Autodesk Inventor part; units mm, degrees
(part 2 of 4)
  arc A616 (35.0017, 10.0056) -> (35.1102, 10.39) centre (15.3265, 15.7621) ccw
  arc A617 (35.3927, 11.567) -> (35.4707, 11.9588) centre (15.3265, 15.7621) ccw
  arc A618 (35.66, 13.1543) -> (35.707, 13.551) centre (15.3265, 15.7621) ccw
  arc A619 (35.8019, 14.7577) -> (35.8176, 15.1569) centre (15.3265, 15.7621) ccw
  arc A620 (35.8176, 16.3673) -> (35.8019, 16.7664) centre (15.3265, 15.7621) ccw
  arc A621 (35.707, 17.9731) -> (35.66, 18.3698) centre (15.3265, 15.7621) ccw
  arc A622 (35.4707, 19.5653) -> (35.3927, 19.9571) centre (15.3265, 15.7621) ccw
  arc A623 (35.1102, 21.1341) -> (35.0017, 21.5186) centre (15.3265, 15.7621) ccw
  arc A624 (34.6277, 22.6697) -> (34.4894, 23.0445) centre (15.3265, 15.7621) ccw
  arc A625 (34.0262, 24.1628) -> (33.859, 24.5256) centre (15.3265, 15.7621) ccw
  arc A626 (33.3095, 25.6041) -> (33.1143, 25.9526) centre (15.3265, 15.7621) ccw
  arc A627 (32.4818, 26.9846) -> (32.2599, 27.3168) centre (15.3265, 15.7621) ccw
  arc A628 (31.5484, 28.296) -> (31.3011, 28.6097) centre (15.3265, 15.7621) ccw
  arc A629 (30.515, 29.5302) -> (30.2439, 29.8235) centre (15.3265, 15.7621) ccw
  arc A630 (29.388, 30.6794) -> (29.0946, 30.9505) centre (15.3265, 15.7621) ccw
  arc A631 (28.1742, 31.7366) -> (27.8605, 31.984) centre (15.3265, 15.7621) ccw
  arc A632 (26.8813, 32.6954) -> (26.5491, 32.9173) centre (15.3265, 15.7621) ccw
  arc A633 (25.5171, 33.5498) -> (25.1685, 33.745) centre (15.3265, 15.7621) ccw
  arc A634 (24.09, 34.2945) -> (23.7273, 34.4617) centre (15.3265, 15.7621) ccw
  arc A635 (22.609, 34.9249) -> (22.2342, 35.0632) centre (15.3265, 15.7621) ccw
  arc A636 (21.083, 35.4372) -> (20.6986, 35.5457) centre (15.3265, 15.7621) ccw
  arc A637 (19.5216, 35.8282) -> (19.1298, 35.9062) centre (15.3265, 15.7621) ccw
  arc A638 (17.9343, 36.0955) -> (17.5376, 36.1425) centre (15.3265, 15.7621) ccw
  arc A639 (16.3309, 36.2374) -> (15.9318, 36.2531) centre (15.3265, 15.7621) ccw
  line L0 (-7.1735, 15.7621) -> (37.8265, 15.7621)
  line L1 (15.3265, -6.7379) -> (15.3265, 38.2621)
  point P0 (0, 0)
  constraints: 960 point on circle, 480 centre point, 4 end point, 2 horizontal alignment, 2 vertical alignment, 476 other
extrude "押し出し1" add sketch "スケッチ1" along normal blind 3
sketch "スケッチ2" plane through (0, 0, 3) normal (0, 0, 1) x (1, 0, 0)
  arc A0 (15.6046, 35.4366) -> (15.5162, 35.1361) centre (20.6157, 33.7992) ccw
  arc A1 (15.5162, 35.1361) -> (15.1369, 35.1361) centre (15.3265, 15.7621) ccw
  arc A2 (15.1369, 35.1361) -> (15.0485, 35.4366) centre (10.0373, 33.7992) ccw
  arc A3 (15.0485, 35.4366) -> (14.9147, 35.8071) centre (8.9575, 33.447) ccw
  arc A4 (14.9147, 35.8071) -> (14.7213, 36.2531) centre (7.8607, 33.0129) ccw
  arc A5 (14.7213, 36.2531) -> (14.3222, 36.2374) centre (15.3265, 15.7621) ccw
  arc A6 (14.3222, 36.2374) -> (14.1644, 35.7777) centre (21.4159, 33.5455) ccw
  arc A7 (14.1644, 35.7777) -> (14.0601, 35.3977) centre (20.2884, 33.8922) ccw
  arc A8 (14.0601, 35.3977) -> (13.9955, 35.0913) centre (19.1843, 34.1586) ccw
  arc A9 (13.9955, 35.0913) -> (13.6174, 35.0615) centre (15.3265, 15.7621) ccw
  arc A10 (13.6174, 35.0615) -> (13.5057, 35.3541) centre (8.6385, 33.3286) ccw
  arc A11 (13.5057, 35.3541) -> (13.3433, 35.713) centre (7.5896, 32.8927) ccw
  arc A12 (13.3433, 35.713) -> (13.1155, 36.1425) centre (6.5302, 32.3739) ccw
  arc A13 (13.1155, 36.1425) -> (12.7188, 36.0955) centre (15.3265, 15.7621) ccw
  arc A14 (12.7188, 36.0955) -> (12.5975, 35.6248) centre (20.0019, 33.9684) ccw
  arc A15 (12.5975, 35.6248) -> (12.5234, 35.2378) centre (18.8506, 34.2256) ccw
  arc A16 (12.5234, 35.2378) -> (12.4831, 34.9273) centre (17.729, 34.4045) ccw
  arc A17 (12.4831, 34.9273) -> (12.1085, 34.8679) centre (15.3265, 15.7621) ccw
  arc A18 (12.1085, 34.8679) -> (11.9742, 35.1509) centre (7.2808, 32.7497) ccw
  arc A19 (11.9742, 35.1509) -> (11.7841, 35.4959) centre (6.2694, 32.2329) ccw
  arc A20 (11.7841, 35.4959) -> (11.5233, 35.9062) centre (5.254, 31.6326) ccw
  arc A21 (11.5233, 35.9062) -> (11.1315, 35.8282) centre (15.3265, 15.7621) ccw
  arc A22 (11.1315, 35.8282) -> (11.0475, 35.3494) centre (18.559, 34.2791) ccw
  arc A23 (11.0475, 35.3494) -> (11.0039, 34.9579) centre (17.3911, 34.4452) ccw
  arc A24 (11.0039, 34.9579) -> (10.9881, 34.6451) centre (16.2589, 34.5355) ccw
  arc A25 (10.9881, 34.6451) -> (10.6194, 34.5566) centre (15.3265, 15.7621) ccw
  arc A26 (10.6194, 34.5566) -> (10.4633, 34.8281) centre (5.9728, 32.0661) ccw
  arc A27 (10.4633, 34.8281) -> (10.2467, 35.1572) centre (5.005, 31.4715) ccw
  arc A28 (10.2467, 35.1572) -> (9.9545, 35.5457) centre (4.0399, 30.7934) ccw
  arc A29 (9.9545, 35.5457) -> (9.57, 35.4372) centre (15.3265, 15.7621) ccw
  arc A30 (9.57, 35.4372) -> (9.5239, 34.9533) centre (17.0962, 34.4756) ccw
  arc A31 (9.5239, 34.9533) -> (9.5112, 34.5595) centre (15.9189, 34.5495) ccw
  arc A32 (9.5112, 34.5595) -> (9.52, 34.2465) centre (14.7831, 34.5508) ccw
  arc A33 (9.52, 34.2465) -> (9.1593, 34.1293) centre (15.3265, 15.7621) ccw
  arc A34 (9.1593, 34.1293) -> (8.9824, 34.3877) centre (4.7224, 31.2819) ccw
  arc A35 (8.9824, 34.3877) -> (8.7406, 34.6988) centre (3.8043, 30.6133) ccw
  arc A36 (8.7406, 34.6988) -> (8.4189, 35.0632) centre (2.8953, 29.8615) ccw
  arc A37 (8.4189, 35.0632) -> (8.0441, 34.9249) centre (15.3265, 15.7621) ccw
  arc A38 (8.0441, 34.9249) -> (8.0361, 34.4389) centre (15.6225, 34.5568) ccw
  arc A39 (8.0361, 34.4389) -> (8.0543, 34.0453) centre (14.443, 34.5381) ccw
  arc A40 (8.0543, 34.0453) -> (8.0876, 33.7339) centre (13.3106, 34.4503) ccw
  arc A41 (8.0876, 33.7339) -> (7.7372, 33.5888) centre (15.3265, 15.7621) ccw
  arc A42 (7.7372, 33.5888) -> (7.5406, 33.8326) centre (3.5375, 30.4021) ccw
  arc A43 (7.5406, 33.8326) -> (7.2752, 34.1237) centre (2.6746, 29.6635) ccw
  arc A44 (7.2752, 34.1237) -> (6.9258, 34.4617) centre (1.8274, 28.8427) ccw
  arc A45 (6.9258, 34.4617) -> (6.563, 34.2945) centre (15.3265, 15.7621) ccw
  arc A46 (6.563, 34.2945) -> (6.5932, 33.8093) centre (14.147, 34.5221) ccw
  arc A47 (6.5932, 33.8093) -> (6.6422, 33.4184) centre (12.9726, 34.4109) ccw
  arc A48 (6.6422, 33.4184) -> (6.6999, 33.1106) centre (11.8506, 34.2345) ccw
  arc A49 (6.6999, 33.1106) -> (6.3619, 32.9384) centre (15.3265, 15.7621) ccw
  arc A50 (6.3619, 32.9384) -> (6.1468, 33.166) centre (2.4252, 29.432) ccw
  arc A51 (6.1468, 33.166) -> (5.8594, 33.4354) centre (1.6229, 28.628) ccw
  arc A52 (5.8594, 33.4354) -> (5.4845, 33.745) centre (0.8427, 27.7432) ccw
  arc A53 (5.4845, 33.745) -> (5.136, 33.5498) centre (15.3265, 15.7621) ccw
  arc A54 (5.136, 33.5498) -> (5.2041, 33.0685) centre (12.6787, 34.3717) ccw
  arc A55 (5.2041, 33.0685) -> (5.2837, 32.6826) centre (11.5167, 34.1687) ccw
  arc A56 (5.2837, 32.6826) -> (5.3653, 32.3803) centre (10.412, 33.9048) ccw
  arc A57 (5.3653, 32.3803) -> (5.0419, 32.1821) centre (15.3265, 15.7621) ccw
  arc A58 (5.0419, 32.1821) -> (4.8096, 32.3921) centre (1.3924, 28.3776) ccw
  arc A59 (4.8096, 32.3921) -> (4.5019, 32.6381) centre (0.6557, 27.5131) ccw
  arc A60 (4.5019, 32.6381) -> (4.104, 32.9173) centre (-0.0527, 26.5699) ccw
  arc A61 (4.104, 32.9173) -> (3.7718, 32.6954) centre (15.3265, 15.7621) ccw
  arc A62 (3.7718, 32.6954) -> (3.8775, 32.2209) centre (11.2268, 34.1066) ccw
  arc A63 (3.8775, 32.2209) -> (3.9871, 31.8425) centre (10.0843, 33.8131) ccw
  arc A64 (3.9871, 31.8425) -> (4.0922, 31.5475) centre (9.0037, 33.4633) ccw
  arc A65 (4.0922, 31.5475) -> (3.7853, 31.3246) centre (15.3265, 15.7621) ccw
  arc A66 (3.7853, 31.3246) -> (3.5372, 31.5157) centre (0.4455, 27.2455) ccw
  arc A67 (3.5372, 31.5157) -> (3.2112, 31.7368) centre (-0.221, 26.3258) ccw
  arc A68 (3.2112, 31.7368) -> (2.7926, 31.984) centre (-0.8532, 25.33) ccw
  arc A69 (2.7926, 31.984) -> (2.4789, 31.7366) centre (15.3265, 15.7621) ccw
  arc A70 (2.4789, 31.7366) -> (2.6214, 31.2719) centre (9.8001, 33.7284) ccw
  arc A71 (2.6214, 31.2719) -> (2.7604, 30.9032) centre (8.6842, 33.3461) ccw
  arc A72 (2.7604, 30.9032) -> (2.8883, 30.6174) centre (7.6343, 32.9126) ccw
  arc A73 (2.8883, 30.6174) -> (2.5999, 30.3711) centre (15.3265, 15.7621) ccw
  arc A74 (2.5999, 30.3711) -> (2.3376, 30.5421) centre (-0.4096, 26.0425) ccw
  arc A75 (2.3376, 30.5421) -> (1.9952, 30.737) centre (-1.0019, 25.0734) ccw
  arc A76 (1.9952, 30.737) -> (1.5585, 30.9505) centre (-1.554, 24.031) ccw
  arc A77 (1.5585, 30.9505) -> (1.2651, 30.6794) centre (15.3265, 15.7621) ccw
  arc A78 (1.2651, 30.6794) -> (1.4437, 30.2273) centre (8.4075, 33.2394) ccw
  arc A79 (1.4437, 30.2273) -> (1.6111, 29.8706) centre (7.325, 32.7708) ccw
  arc A80 (1.6111, 29.8706) -> (1.7611, 29.5957) centre (6.3124, 32.2563) ccw
  arc A81 (1.7611, 29.5957) -> (1.4929, 29.3275) centre (15.3265, 15.7621) ccw
  arc A82 (1.4929, 29.3275) -> (1.218, 29.4775) centre (-1.1676, 24.7762) ccw
  arc A83 (1.218, 29.4775) -> (0.8613, 29.6449) centre (-1.6821, 23.7636) ccw
  arc A84 (0.8613, 29.6449) -> (0.4092, 29.8235) centre (-2.1508, 22.6811) ccw
  arc A85 (0.4092, 29.8235) -> (0.1381, 29.5302) centre (15.3265, 15.7621) ccw
  arc A86 (0.1381, 29.5302) -> (0.3516, 29.0934) centre (7.0576, 32.6427) ccw
  arc A87 (0.3516, 29.0934) -> (0.5465, 28.751) centre (6.0152, 32.0905) ccw
  arc A88 (0.5465, 28.751) -> (0.7175, 28.4887) centre (5.0461, 31.4982) ccw
  arc A89 (0.7175, 28.4887) -> (0.4712, 28.2003) centre (15.3265, 15.7621) ccw
  arc A90 (0.4712, 28.2003) -> (0.1854, 28.3282) centre (-1.824, 23.4543) ccw
  arc A91 (0.1854, 28.3282) -> (-0.1833, 28.4672) centre (-2.2575, 22.4045) ccw
  arc A92 (-0.1833, 28.4672) -> (-0.648, 28.6097) centre (-2.6398, 21.2885) ccw
  arc A93 (-0.648, 28.6097) -> (-0.8953, 28.296) centre (15.3265, 15.7621) ccw
  arc A94 (-0.8953, 28.296) -> (-0.6482, 27.8774) centre (5.7587, 31.9418) ccw
  arc A95 (-0.6482, 27.8774) -> (-0.4271, 27.5514) centre (4.7628, 31.3096) ccw
  arc A96 (-0.4271, 27.5514) -> (-0.236, 27.3033) centre (3.8431, 30.6431) ccw
  arc A97 (-0.236, 27.3033) -> (-0.4589, 26.9964) centre (15.3265, 15.7621) ccw
  arc A98 (-0.4589, 26.9964) -> (-0.7539, 27.1015) centre (-2.3747, 22.085) ccw
  arc A99 (-0.7539, 27.1015) -> (-1.1323, 27.2111) centre (-2.7245, 21.0044) ccw
  arc A100 (-1.1323, 27.2111) -> (-1.6068, 27.3168) centre (-3.018, 19.8618) ccw
  arc A101 (-1.6068, 27.3168) -> (-1.8287, 26.9846) centre (15.3265, 15.7621) ccw
  arc A102 (-1.8287, 26.9846) -> (-1.5495, 26.5867) centre (4.5187, 31.1413) ccw
  arc A103 (-1.5495, 26.5867) -> (-1.3035, 26.279) centre (3.5755, 30.4329) ccw
  arc A104 (-1.3035, 26.279) -> (-1.0935, 26.0467) centre (2.711, 29.6962) ccw
  arc A105 (-1.0935, 26.0467) -> (-1.2916, 25.7233) centre (15.3265, 15.7621) ccw
  arc A106 (-1.2916, 25.7233) -> (-1.594, 25.8049) centre (-2.8162, 20.6766) ccw
  arc A107 (-1.594, 25.8049) -> (-1.9799, 25.8845) centre (-3.0801, 19.5719) ccw
  arc A108 (-1.9799, 25.8845) -> (-2.4612, 25.9526) centre (-3.2831, 18.4099) ccw
  arc A109 (-2.4612, 25.9526) -> (-2.6564, 25.6041) centre (15.3265, 15.7621) ccw
  arc A110 (-2.6564, 25.6041) -> (-2.3468, 25.2293) centre (3.3454, 30.2459) ccw
  arc A111 (-2.3468, 25.2293) -> (-2.0774, 24.9418) centre (2.4606, 29.4657) ccw
  arc A112 (-2.0774, 24.9418) -> (-1.8498, 24.7267) centre (1.6566, 28.6635) ccw
  arc A113 (-1.8498, 24.7267) -> (-2.022, 24.3888) centre (15.3265, 15.7621) ccw
  arc A114 (-2.022, 24.3888) -> (-2.3298, 24.4464) centre (-3.1459, 19.238) ccw
  arc A115 (-2.3298, 24.4464) -> (-2.7207, 24.4954) centre (-3.3223, 18.116) ccw
  arc A116 (-2.7207, 24.4954) -> (-3.2059, 24.5256) centre (-3.4335, 16.9417) ccw
  arc A117 (-3.2059, 24.5256) -> (-3.3731, 24.1628) centre (15.3265, 15.7621) ccw
  arc A118 (-3.3731, 24.1628) -> (-3.0351, 23.8134) centre (2.2459, 29.2612) ccw
  arc A119 (-3.0351, 23.8134) -> (-2.7439, 23.548) centre (1.4251, 28.414) ccw
  arc A120 (-2.7439, 23.548) -> (-2.5002, 23.3514) centre (0.6865, 27.5512) ccw
  arc A121 (-2.5002, 23.3514) -> (-2.6453, 23.001) centre (15.3265, 15.7621) ccw
  arc A122 (-2.6453, 23.001) -> (-2.9567, 23.0343) centre (-3.3617, 17.778) ccw
  arc A123 (-2.9567, 23.0343) -> (-3.3503, 23.0525) centre (-3.4495, 16.6456) ccw
  arc A124 (-3.3503, 23.0525) -> (-3.8363, 23.0445) centre (-3.4682, 15.4661) ccw
  arc A125 (-3.8363, 23.0445) -> (-3.9746, 22.6697) centre (15.3265, 15.7621) ccw
  arc A126 (-3.9746, 22.6697) -> (-3.6102, 22.348) centre (1.2271, 28.1933) ccw
  arc A127 (-3.6102, 22.348) -> (-3.2991, 22.1062) centre (0.4753, 27.2843) ccw
  arc A128 (-3.2991, 22.1062) -> (-3.0407, 21.9293) centre (-0.1933, 26.3662) ccw
  arc A129 (-3.0407, 21.9293) -> (-3.1579, 21.5686) centre (15.3265, 15.7621) ccw
  arc A130 (-3.1579, 21.5686) -> (-3.4709, 21.5774) centre (-3.4622, 16.3055) ccw
  arc A131 (-3.4709, 21.5774) -> (-3.8647, 21.5647) centre (-3.4609, 15.1697) ccw
  arc A132 (-3.8647, 21.5647) -> (-4.3486, 21.5186) centre (-3.387, 13.9924) ccw
  arc A133 (-4.3486, 21.5186) -> (-4.4571, 21.1341) centre (15.3265, 15.7621) ccw
  arc A134 (-4.4571, 21.1341) -> (-4.0686, 20.8419) centre (0.2952, 27.0488) ccw
  arc A135 (-4.0686, 20.8419) -> (-3.7395, 20.6253) centre (-0.3829, 26.0836) ccw
  arc A136 (-3.7395, 20.6253) -> (-3.468, 20.4692) centre (-0.9775, 25.1158) ccw
  arc A137 (-3.468, 20.4692) -> (-3.5565, 20.1005) centre (15.3265, 15.7621) ccw
  arc A138 (-3.5565, 20.1005) -> (-3.8693, 20.0847) centre (-3.4469, 14.8297) ccw
  arc A139 (-3.8693, 20.0847) -> (-4.2608, 20.0411) centre (-3.3565, 13.6975) ccw
  arc A140 (-4.2608, 20.0411) -> (-4.7396, 19.9571) centre (-3.1905, 12.5296) ccw
  arc A141 (-4.7396, 19.9571) -> (-4.8176, 19.5653) centre (15.3265, 15.7621) ccw
  arc A142 (-4.8176, 19.5653) -> (-4.4073, 19.3045) centre (-0.544, 25.8346) ccw
  arc A143 (-4.4073, 19.3045) -> (-4.0622, 19.1144) centre (-1.1443, 24.8192) ccw
  arc A144 (-4.0622, 19.1144) -> (-3.7793, 18.9801) centre (-1.6611, 23.8078) ccw
  arc A145 (-3.7793, 18.9801) -> (-3.8387, 18.6055) centre (15.3265, 15.7621) ccw
  arc A146 (-3.8387, 18.6055) -> (-4.1492, 18.5653) centre (-3.3159, 13.3596) ccw
  arc A147 (-4.1492, 18.5653) -> (-4.5362, 18.4911) centre (-3.137, 12.238) ccw
  arc A148 (-4.5362, 18.4911) -> (-5.0069, 18.3698) centre (-2.8798, 11.0868) ccw
  arc A149 (-5.0069, 18.3698) -> (-5.0539, 17.9731) centre (15.3265, 15.7621) ccw
  arc A150 (-5.0539, 17.9731) -> (-4.6244, 17.7453) centre (-1.2853, 24.5584) ccw
  arc A151 (-4.6244, 17.7453) -> (-4.2655, 17.5829) centre (-1.8041, 23.499) ccw
  arc A152 (-4.2655, 17.5829) -> (-3.9729, 17.4712) centre (-2.24, 22.4501) ccw
  arc A153 (-3.9729, 17.4712) -> (-4.0027, 17.0931) centre (15.3265, 15.7621) ccw
  arc A154 (-4.0027, 17.0931) -> (-4.3091, 17.0286) centre (-3.0699, 11.9043) ccw
  arc A155 (-4.3091, 17.0286) -> (-4.6891, 16.9243) centre (-2.8036, 10.8002) ccw
  arc A156 (-4.6891, 16.9243) -> (-5.1488, 16.7664) centre (-2.4569, 9.6727) ccw
  arc A157 (-5.1488, 16.7664) -> (-5.1645, 16.3673) centre (15.3265, 15.7621) ccw
  arc A158 (-5.1645, 16.3673) -> (-4.7185, 16.1739) centre (-1.9243, 23.2279) ccw
  arc A159 (-4.7185, 16.1739) -> (-4.348, 16.0401) centre (-2.3584, 22.1311) ccw
  arc A160 (-4.348, 16.0401) -> (-4.0475, 15.9517) centre (-2.7106, 21.0513) ccw
  arc A161 (-4.0475, 15.9517) -> (-4.0475, 15.5724) centre (15.3265, 15.7621) ccw
  arc A162 (-4.0475, 15.5724) -> (-4.348, 15.4841) centre (-2.7106, 10.4729) ccw
  arc A163 (-4.348, 15.4841) -> (-4.7185, 15.3503) centre (-2.3584, 9.3931) ccw
  arc A164 (-4.7185, 15.3503) -> (-5.1645, 15.1569) centre (-1.9243, 8.2962) ccw
  arc A165 (-5.1645, 15.1569) -> (-5.1488, 14.7577) centre (15.3265, 15.7621) ccw
  arc A166 (-5.1488, 14.7577) -> (-4.6891, 14.5999) centre (-2.4569, 21.8514) ccw
  arc A167 (-4.6891, 14.5999) -> (-4.3091, 14.4956) centre (-2.8036, 20.7239) ccw
  arc A168 (-4.3091, 14.4956) -> (-4.0027, 14.431) centre (-3.0699, 19.6198) ccw
  arc A169 (-4.0027, 14.431) -> (-3.9729, 14.053) centre (15.3265, 15.7621) ccw
  arc A170 (-3.9729, 14.053) -> (-4.2655, 13.9413) centre (-2.24, 9.074) ccw
  arc A171 (-4.2655, 13.9413) -> (-4.6244, 13.7788) centre (-1.8041, 8.0251) ccw
  arc A172 (-4.6244, 13.7788) -> (-5.0539, 13.551) centre (-1.2853, 6.9657) ccw
  arc A173 (-5.0539, 13.551) -> (-5.0069, 13.1543) centre (15.3265, 15.7621) ccw
  arc A174 (-5.0069, 13.1543) -> (-4.5362, 13.033) centre (-2.8798, 20.4374) ccw
  arc A175 (-4.5362, 13.033) -> (-4.1492, 12.9589) centre (-3.137, 19.2861) ccw
  arc A176 (-4.1492, 12.9589) -> (-3.8387, 12.9186) centre (-3.3159, 18.1645) ccw
  arc A177 (-3.8387, 12.9186) -> (-3.7793, 12.544) centre (15.3265, 15.7621) ccw
  arc A178 (-3.7793, 12.544) -> (-4.0622, 12.4097) centre (-1.6611, 7.7164) ccw
  arc A179 (-4.0622, 12.4097) -> (-4.4073, 12.2196) centre (-1.1443, 6.7049) ccw
  arc A180 (-4.4073, 12.2196) -> (-4.8176, 11.9588) centre (-0.544, 5.6895) ccw
  arc A181 (-4.8176, 11.9588) -> (-4.7396, 11.567) centre (15.3265, 15.7621) ccw
  arc A182 (-4.7396, 11.567) -> (-4.2608, 11.4831) centre (-3.1905, 18.9945) ccw
  arc A183 (-4.2608, 11.4831) -> (-3.8693, 11.4395) centre (-3.3565, 17.8266) ccw
  arc A184 (-3.8693, 11.4395) -> (-3.5565, 11.4237) centre (-3.4469, 16.6945) ccw
  arc A185 (-3.5565, 11.4237) -> (-3.468, 11.0549) centre (15.3265, 15.7621) ccw
  arc A186 (-3.468, 11.0549) -> (-3.7395, 10.8988) centre (-0.9775, 6.4083) ccw
  arc A187 (-3.7395, 10.8988) -> (-4.0686, 10.6822) centre (-0.3829, 5.4406) ccw
  arc A188 (-4.0686, 10.6822) -> (-4.4571, 10.39) centre (0.2952, 4.4754) ccw
  arc A189 (-4.4571, 10.39) -> (-4.3486, 10.0056) centre (15.3265, 15.7621) ccw
  arc A190 (-4.3486, 10.0056) -> (-3.8647, 9.9594) centre (-3.387, 17.5317) ccw
  arc A191 (-3.8647, 9.9594) -> (-3.4709, 9.9467) centre (-3.4609, 16.3544) ccw
  arc A192 (-3.4709, 9.9467) -> (-3.1579, 9.9555) centre (-3.4622, 15.2186) ccw
  arc A193 (-3.1579, 9.9555) -> (-3.0407, 9.5948) centre (15.3265, 15.7621) ccw
  arc A194 (-3.0407, 9.5948) -> (-3.2991, 9.4179) centre (-0.1933, 5.158) ccw
  arc A195 (-3.2991, 9.4179) -> (-3.6102, 9.1762) centre (0.4753, 4.2398) ccw
  arc A196 (-3.6102, 9.1762) -> (-3.9746, 8.8544) centre (1.2271, 3.3308) ccw
  arc A197 (-3.9746, 8.8544) -> (-3.8363, 8.4796) centre (15.3265, 15.7621) ccw
  arc A198 (-3.8363, 8.4796) -> (-3.3503, 8.4716) centre (-3.4682, 16.058) ccw
  arc A199 (-3.3503, 8.4716) -> (-2.9567, 8.4898) centre (-3.4495, 14.8785) ccw
  arc A200 (-2.9567, 8.4898) -> (-2.6453, 8.5231) centre (-3.3617, 13.7462) ccw
  arc A201 (-2.6453, 8.5231) -> (-2.5002, 8.1727) centre (15.3265, 15.7621) ccw
  arc A202 (-2.5002, 8.1727) -> (-2.7439, 7.9761) centre (0.6865, 3.973) ccw
  arc A203 (-2.7439, 7.9761) -> (-3.0351, 7.7107) centre (1.4251, 3.1101) ccw
  arc A204 (-3.0351, 7.7107) -> (-3.3731, 7.3613) centre (2.2459, 2.2629) ccw
  arc A205 (-3.3731, 7.3613) -> (-3.2059, 6.9986) centre (15.3265, 15.7621) ccw
  arc A206 (-3.2059, 6.9986) -> (-2.7207, 7.0287) centre (-3.4335, 14.5825) ccw
  arc A207 (-2.7207, 7.0287) -> (-2.3298, 7.0777) centre (-3.3223, 13.4081) ccw
  arc A208 (-2.3298, 7.0777) -> (-2.022, 7.1354) centre (-3.1459, 12.2861) ccw
  arc A209 (-2.022, 7.1354) -> (-1.8498, 6.7975) centre (15.3265, 15.7621) ccw
  arc A210 (-1.8498, 6.7975) -> (-2.0774, 6.5823) centre (1.6566, 2.8607) ccw
  arc A211 (-2.0774, 6.5823) -> (-2.3468, 6.2949) centre (2.4606, 2.0585) ccw
  arc A212 (-2.3468, 6.2949) -> (-2.6564, 5.9201) centre (3.3454, 1.2782) ccw
  arc A213 (-2.6564, 5.9201) -> (-2.4612, 5.5715) centre (15.3265, 15.7621) ccw
  arc A214 (-2.4612, 5.5715) -> (-1.9799, 5.6397) centre (-3.2831, 13.1142) ccw
  arc A215 (-1.9799, 5.6397) -> (-1.594, 5.7192) centre (-3.0801, 11.9522) ccw
  arc A216 (-1.594, 5.7192) -> (-1.2916, 5.8008) centre (-2.8162, 10.8475) ccw
  arc A217 (-1.2916, 5.8008) -> (-1.0935, 5.4775) centre (15.3265, 15.7621) ccw
  arc A218 (-1.0935, 5.4775) -> (-1.3035, 5.2451) centre (2.711, 1.8279) ccw
  arc A219 (-1.3035, 5.2451) -> (-1.5495, 4.9374) centre (3.5755, 1.0913) ccw
  arc A220 (-1.5495, 4.9374) -> (-1.8287, 4.5395) centre (4.5187, 0.3829) ccw
  arc A221 (-1.8287, 4.5395) -> (-1.6068, 4.2073) centre (15.3265, 15.7621) ccw
  arc A222 (-1.6068, 4.2073) -> (-1.1323, 4.313) centre (-3.018, 11.6623) ccw
  arc A223 (-1.1323, 4.313) -> (-0.7539, 4.4226) centre (-2.7245, 10.5198) ccw
  arc A224 (-0.7539, 4.4226) -> (-0.4589, 4.5277) centre (-2.3747, 9.4392) ccw
  arc A225 (-0.4589, 4.5277) -> (-0.236, 4.2209) centre (15.3265, 15.7621) ccw
  arc A226 (-0.236, 4.2209) -> (-0.4271, 3.9728) centre (3.8431, 0.8811) ccw
  arc A227 (-0.4271, 3.9728) -> (-0.6482, 3.6467) centre (4.7628, 0.2145) ccw
  arc A228 (-0.6482, 3.6467) -> (-0.8953, 3.2281) centre (5.7587, -0.4177) ccw
  arc A229 (-0.8953, 3.2281) -> (-0.648, 2.9144) centre (15.3265, 15.7621) ccw
  arc A230 (-0.648, 2.9144) -> (-0.1833, 3.057) centre (-2.6398, 10.2356) ccw
  arc A231 (-0.1833, 3.057) -> (0.1854, 3.1959) centre (-2.2575, 9.1197) ccw
  arc A232 (0.1854, 3.1959) -> (0.4712, 3.3238) centre (-1.824, 8.0698) ccw
  arc A233 (0.4712, 3.3238) -> (0.7175, 3.0354) centre (15.3265, 15.7621) ccw
  arc A234 (0.7175, 3.0354) -> (0.5465, 2.7731) centre (5.0461, 0.026) ccw
  arc A235 (0.5465, 2.7731) -> (0.3516, 2.4307) centre (6.0152, -0.5664) ccw
  arc A236 (0.3516, 2.4307) -> (0.1381, 1.994) centre (7.0576, -1.1185) ccw
  arc A237 (0.1381, 1.994) -> (0.4092, 1.7006) centre (15.3265, 15.7621) ccw
  arc A238 (0.4092, 1.7006) -> (0.8613, 1.8792) centre (-2.1508, 8.843) ccw
  arc A239 (0.8613, 1.8792) -> (1.218, 2.0467) centre (-1.6821, 7.7605) ccw
  arc A240 (1.218, 2.0467) -> (1.4929, 2.1966) centre (-1.1676, 6.7479) ccw
  arc A241 (1.4929, 2.1966) -> (1.7611, 1.9284) centre (15.3265, 15.7621) ccw
  arc A242 (1.7611, 1.9284) -> (1.6111, 1.6535) centre (6.3124, -0.7321) ccw
  arc A243 (1.6111, 1.6535) -> (1.4437, 1.2969) centre (7.325, -1.2466) ccw
  arc A244 (1.4437, 1.2969) -> (1.2651, 0.8447) centre (8.4075, -1.7153) ccw
  arc A245 (1.2651, 0.8447) -> (1.5585, 0.5736) centre (15.3265, 15.7621) ccw
  arc A246 (1.5585, 0.5736) -> (1.9952, 0.7871) centre (-1.554, 7.4931) ccw
  arc A247 (1.9952, 0.7871) -> (2.3376, 0.982) centre (-1.0019, 6.4507) ccw
  arc A248 (2.3376, 0.982) -> (2.5999, 1.1531) centre (-0.4096, 5.4816) ccw
  arc A249 (2.5999, 1.1531) -> (2.8883, 0.9068) centre (15.3265, 15.7621) ccw
  arc A250 (2.8883, 0.9068) -> (2.7604, 0.6209) centre (7.6343, -1.3885) ccw
  arc A251 (2.7604, 0.6209) -> (2.6214, 0.2522) centre (8.6842, -1.822) ccw
  arc A252 (2.6214, 0.2522) -> (2.4789, -0.2125) centre (9.8001, -2.2042) ccw
  arc A253 (2.4789, -0.2125) -> (2.7926, -0.4598) centre (15.3265, 15.7621) ccw
  arc A254 (2.7926, -0.4598) -> (3.2112, -0.2127) centre (-0.8532, 6.1942) ccw
  arc A255 (3.2112, -0.2127) -> (3.5372, 0.0085) centre (-0.221, 5.1983) ccw
  arc A256 (3.5372, 0.0085) -> (3.7853, 0.1996) centre (0.4455, 4.2787) ccw
  arc A257 (3.7853, 0.1996) -> (4.0922, -0.0233) centre (15.3265, 15.7621) ccw
  arc A258 (4.0922, -0.0233) -> (3.9871, -0.3184) centre (9.0037, -1.9392) ccw
  arc A259 (3.9871, -0.3184) -> (3.8775, -0.6968) centre (10.0843, -2.2889) ccw
  arc A260 (3.8775, -0.6968) -> (3.7718, -1.1713) centre (11.2268, -2.5825) ccw
  arc A261 (3.7718, -1.1713) -> (4.104, -1.3932) centre (15.3265, 15.7621) ccw
  arc A262 (4.104, -1.3932) -> (4.5019, -1.114) centre (-0.0527, 4.9542) ccw
  arc A263 (4.5019, -1.114) -> (4.8096, -0.868) centre (0.6557, 4.011) ccw
  arc A264 (4.8096, -0.868) -> (5.0419, -0.658) centre (1.3924, 3.1465) ccw
  arc A265 (5.0419, -0.658) -> (5.3653, -0.8561) centre (15.3265, 15.7621) ccw
  arc A266 (5.3653, -0.8561) -> (5.2837, -1.1585) centre (10.412, -2.3807) ccw
  arc A267 (5.2837, -1.1585) -> (5.2041, -1.5443) centre (11.5167, -2.6446) ccw
  arc A268 (5.2041, -1.5443) -> (5.136, -2.0257) centre (12.6787, -2.8476) ccw
  arc A269 (5.136, -2.0257) -> (5.4845, -2.2208) centre (15.3265, 15.7621) ccw
  arc A270 (5.4845, -2.2208) -> (5.8594, -1.9113) centre (0.8427, 3.7809) ccw
  arc A271 (5.8594, -1.9113) -> (6.1468, -1.6418) centre (1.6229, 2.8962) ccw
  arc A272 (6.1468, -1.6418) -> (6.3619, -1.4143) centre (2.4252, 2.0921) ccw
  arc A273 (6.3619, -1.4143) -> (6.6999, -1.5864) centre (15.3265, 15.7621) ccw
  arc A274 (6.6999, -1.5864) -> (6.6422, -1.8943) centre (11.8506, -2.7104) ccw
  arc A275 (6.6422, -1.8943) -> (6.5932, -2.2852) centre (12.9726, -2.8868) ccw
  arc A276 (6.5932, -2.2852) -> (6.563, -2.7704) centre (14.147, -2.998) ccw
  arc A277 (6.563, -2.7704) -> (6.9258, -2.9376) centre (15.3265, 15.7621) ccw
  arc A278 (6.9258, -2.9376) -> (7.2752, -2.5996) centre (1.8274, 2.6814) ccw
  arc A279 (7.2752, -2.5996) -> (7.5406, -2.3084) centre (2.6746, 1.8607) ccw
  arc A280 (7.5406, -2.3084) -> (7.7372, -2.0647) centre (3.5375, 1.122) ccw
  arc A281 (7.7372, -2.0647) -> (8.0876, -2.2098) centre (15.3265, 15.7621) ccw
  arc A282 (8.0876, -2.2098) -> (8.0543, -2.5212) centre (13.3106, -2.9261) ccw
  arc A283 (8.0543, -2.5212) -> (8.0361, -2.9148) centre (14.443, -3.014) ccw
  arc A284 (8.0361, -2.9148) -> (8.0441, -3.4008) centre (15.6225, -3.0327) ccw
  arc A285 (8.0441, -3.4008) -> (8.4189, -3.5391) centre (15.3265, 15.7621) ccw
  arc A286 (8.4189, -3.5391) -> (8.7406, -3.1747) centre (2.8953, 1.6626) ccw
  arc A287 (8.7406, -3.1747) -> (8.9824, -2.8636) centre (3.8043, 0.9109) ccw
  arc A288 (8.9824, -2.8636) -> (9.1593, -2.6052) centre (4.7224, 0.2422) ccw
  arc A289 (9.1593, -2.6052) -> (9.52, -2.7224) centre (15.3265, 15.7621) ccw
  arc A290 (9.52, -2.7224) -> (9.5112, -3.0354) centre (14.7831, -3.0267) ccw
  arc A291 (9.5112, -3.0354) -> (9.5239, -3.4292) centre (15.9189, -3.0254) ccw
  arc A292 (9.5239, -3.4292) -> (9.57, -3.9131) centre (17.0962, -2.9515) ccw
  arc A293 (9.57, -3.9131) -> (9.9545, -4.0215) centre (15.3265, 15.7621) ccw
  arc A294 (9.9545, -4.0215) -> (10.2467, -3.633) centre (4.0399, 0.7308) ccw
  arc A295 (10.2467, -3.633) -> (10.4633, -3.3039) centre (5.005, 0.0526) ccw
  arc A296 (10.4633, -3.3039) -> (10.6194, -3.0324) centre (5.9728, -0.5419) ccw
  arc A297 (10.6194, -3.0324) -> (10.9881, -3.121) centre (15.3265, 15.7621) ccw
  arc A298 (10.9881, -3.121) -> (11.0039, -3.4337) centre (16.2589, -3.0114) ccw
  arc A299 (11.0039, -3.4337) -> (11.0475, -3.8253) centre (17.3911, -2.921) ccw
  arc A300 (11.0475, -3.8253) -> (11.1315, -4.3041) centre (18.559, -2.755) ccw
  arc A301 (11.1315, -4.3041) -> (11.5233, -4.382) centre (15.3265, 15.7621) ccw
  arc A302 (11.5233, -4.382) -> (11.7841, -3.9718) centre (5.254, -0.1085) ccw
  arc A303 (11.7841, -3.9718) -> (11.9742, -3.6267) centre (6.2694, -0.7088) ccw
  arc A304 (11.9742, -3.6267) -> (12.1085, -3.3438) centre (7.2808, -1.2256) ccw
  arc A305 (12.1085, -3.3438) -> (12.4831, -3.4031) centre (15.3265, 15.7621) ccw
  arc A306 (12.4831, -3.4031) -> (12.5234, -3.7137) centre (17.729, -2.8804) ccw
  arc A307 (12.5234, -3.7137) -> (12.5975, -4.1006) centre (18.8506, -2.7014) ccw
  arc A308 (12.5975, -4.1006) -> (12.7188, -4.5714) centre (20.0019, -2.4443) ccw
  arc A309 (12.7188, -4.5714) -> (13.1155, -4.6183) centre (15.3265, 15.7621) ccw
  arc A310 (13.1155, -4.6183) -> (13.3433, -4.1889) centre (6.5302, -0.8498) ccw
  arc A311 (13.3433, -4.1889) -> (13.5057, -3.83) centre (7.5896, -1.3686) ccw
  arc A312 (13.5057, -3.83) -> (13.6174, -3.5374) centre (8.6385, -1.8045) ccw
  arc A313 (13.6174, -3.5374) -> (13.9955, -3.5672) centre (15.3265, 15.7621) ccw
  arc A314 (13.9955, -3.5672) -> (14.0601, -3.8736) centre (19.1843, -2.6344) ccw
  arc A315 (14.0601, -3.8736) -> (14.1644, -4.2535) centre (20.2884, -2.368) ccw
  arc A316 (14.1644, -4.2535) -> (14.3222, -4.7133) centre (21.4159, -2.0213) ccw
  arc A317 (14.3222, -4.7133) -> (14.7213, -4.729) centre (15.3265, 15.7621) ccw
  arc A318 (14.7213, -4.729) -> (14.9147, -4.283) centre (7.8607, -1.4888) ccw
  arc A319 (14.9147, -4.283) -> (15.0485, -3.9124) centre (8.9575, -1.9228) ccw
  arc A320 (15.0485, -3.9124) -> (15.1369, -3.612) centre (10.0373, -2.275) ccw
  arc A321 (15.1369, -3.612) -> (15.5162, -3.612) centre (15.3265, 15.7621) ccw
  arc A322 (15.5162, -3.612) -> (15.6046, -3.9124) centre (20.6157, -2.275) ccw
  arc A323 (15.6046, -3.9124) -> (15.7383, -4.283) centre (21.6956, -1.9228) ccw
  arc A324 (15.7383, -4.283) -> (15.9318, -4.729) centre (22.7924, -1.4888) ccw
  arc A325 (15.9318, -4.729) -> (16.3309, -4.7133) centre (15.3265, 15.7621) ccw
  arc A326 (16.3309, -4.7133) -> (16.4887, -4.2535) centre (9.2372, -2.0213) ccw
  arc A327 (16.4887, -4.2535) -> (16.593, -3.8736) centre (10.3647, -2.368) ccw
  arc A328 (16.593, -3.8736) -> (16.6576, -3.5672) centre (11.4688, -2.6344) ccw
  arc A329 (16.6576, -3.5672) -> (17.0357, -3.5374) centre (15.3265, 15.7621) ccw
  arc A330 (17.0357, -3.5374) -> (17.1473, -3.83) centre (22.0146, -1.8045) ccw
  arc A331 (17.1473, -3.83) -> (17.3098, -4.1889) centre (23.0635, -1.3686) ccw
  arc A332 (17.3098, -4.1889) -> (17.5376, -4.6183) centre (24.1229, -0.8498) ccw
  arc A333 (17.5376, -4.6183) -> (17.9343, -4.5714) centre (15.3265, 15.7621) ccw
  arc A334 (17.9343, -4.5714) -> (18.0556, -4.1006) centre (10.6512, -2.4443) ccw
  arc A335 (18.0556, -4.1006) -> (18.1297, -3.7137) centre (11.8025, -2.7014) ccw
  arc A336 (18.1297, -3.7137) -> (18.17, -3.4031) centre (12.9241, -2.8804) ccw
  arc A337 (18.17, -3.4031) -> (18.5446, -3.3438) centre (15.3265, 15.7621) ccw
  arc A338 (18.5446, -3.3438) -> (18.6789, -3.6267) centre (23.3723, -1.2256) ccw
  arc A339 (18.6789, -3.6267) -> (18.869, -3.9718) centre (24.3837, -0.7088) ccw
  arc A340 (18.869, -3.9718) -> (19.1298, -4.382) centre (25.3991, -0.1085) ccw
  arc A341 (19.1298, -4.382) -> (19.5216, -4.3041) centre (15.3265, 15.7621) ccw
  arc A342 (19.5216, -4.3041) -> (19.6056, -3.8253) centre (12.0941, -2.755) ccw
  arc A343 (19.6056, -3.8253) -> (19.6491, -3.4337) centre (13.262, -2.921) ccw
  arc A344 (19.6491, -3.4337) -> (19.6649, -3.121) centre (14.3942, -3.0114) ccw
  arc A345 (19.6649, -3.121) -> (20.0337, -3.0324) centre (15.3265, 15.7621) ccw
  arc A346 (20.0337, -3.0324) -> (20.1898, -3.3039) centre (24.6803, -0.5419) ccw
  arc A347 (20.1898, -3.3039) -> (20.4064, -3.633) centre (25.648, 0.0526) ccw
  arc A348 (20.4064, -3.633) -> (20.6986, -4.0215) centre (26.6132, 0.7308) ccw
  arc A349 (20.6986, -4.0215) -> (21.083, -3.9131) centre (15.3265, 15.7621) ccw
  arc A350 (21.083, -3.9131) -> (21.1292, -3.4292) centre (13.5569, -2.9515) ccw
  arc A351 (21.1292, -3.4292) -> (21.1419, -3.0354) centre (14.7342, -3.0254) ccw
  arc A352 (21.1419, -3.0354) -> (21.1331, -2.7224) centre (15.87, -3.0267) ccw
  arc A353 (21.1331, -2.7224) -> (21.4938, -2.6052) centre (15.3265, 15.7621) ccw
  arc A354 (21.4938, -2.6052) -> (21.6707, -2.8636) centre (25.9306, 0.2422) ccw
  arc A355 (21.6707, -2.8636) -> (21.9125, -3.1747) centre (26.8488, 0.9109) ccw
  arc A356 (21.9125, -3.1747) -> (22.2342, -3.5391) centre (27.7578, 1.6626) ccw
  arc A357 (22.2342, -3.5391) -> (22.609, -3.4008) centre (15.3265, 15.7621) ccw
  arc A358 (22.609, -3.4008) -> (22.617, -2.9148) centre (15.0306, -3.0327) ccw
  arc A359 (22.617, -2.9148) -> (22.5988, -2.5212) centre (16.2101, -3.014) ccw
  arc A360 (22.5988, -2.5212) -> (22.5655, -2.2098) centre (17.3425, -2.9261) ccw
  arc A361 (22.5655, -2.2098) -> (22.9159, -2.0647) centre (15.3265, 15.7621) ccw
  arc A362 (22.9159, -2.0647) -> (23.1125, -2.3084) centre (27.1156, 1.122) ccw
  arc A363 (23.1125, -2.3084) -> (23.3779, -2.5996) centre (27.9785, 1.8607) ccw
  arc A364 (23.3779, -2.5996) -> (23.7273, -2.9376) centre (28.8257, 2.6814) ccw
  arc A365 (23.7273, -2.9376) -> (24.09, -2.7704) centre (15.3265, 15.7621) ccw
  arc A366 (24.09, -2.7704) -> (24.0599, -2.2852) centre (16.5061, -2.998) ccw
  arc A367 (24.0599, -2.2852) -> (24.0109, -1.8943) centre (17.6805, -2.8868) ccw
  arc A368 (24.0109, -1.8943) -> (23.9532, -1.5864) centre (18.8025, -2.7104) ccw
  arc A369 (23.9532, -1.5864) -> (24.2911, -1.4143) centre (15.3265, 15.7621) ccw
  arc A370 (24.2911, -1.4143) -> (24.5063, -1.6418) centre (28.2279, 2.0921) ccw
  arc A371 (24.5063, -1.6418) -> (24.7937, -1.9113) centre (29.0302, 2.8962) ccw
  arc A372 (24.7937, -1.9113) -> (25.1685, -2.2208) centre (29.8104, 3.7809) ccw
  arc A373 (25.1685, -2.2208) -> (25.5171, -2.0257) centre (15.3265, 15.7621) ccw
  arc A374 (25.5171, -2.0257) -> (25.449, -1.5443) centre (17.9744, -2.8476) ccw
  arc A375 (25.449, -1.5443) -> (25.3694, -1.1585) centre (19.1364, -2.6446) ccw
  arc A376 (25.3694, -1.1585) -> (25.2878, -0.8561) centre (20.2411, -2.3807) ccw
  arc A377 (25.2878, -0.8561) -> (25.6112, -0.658) centre (15.3265, 15.7621) ccw
  arc A378 (25.6112, -0.658) -> (25.8435, -0.868) centre (29.2607, 3.1465) ccw
  arc A379 (25.8435, -0.868) -> (26.1512, -1.114) centre (29.9974, 4.011) ccw
  arc A380 (26.1512, -1.114) -> (26.5491, -1.3932) centre (30.7058, 4.9542) ccw
  arc A381 (26.5491, -1.3932) -> (26.8813, -1.1713) centre (15.3265, 15.7621) ccw
  arc A382 (26.8813, -1.1713) -> (26.7756, -0.6968) centre (19.4263, -2.5825) ccw
  arc A383 (26.7756, -0.6968) -> (26.666, -0.3184) centre (20.5688, -2.2889) ccw
  arc A384 (26.666, -0.3184) -> (26.5609, -0.0233) centre (21.6494, -1.9392) ccw
  arc A385 (26.5609, -0.0233) -> (26.8677, 0.1996) centre (15.3265, 15.7621) ccw
  arc A386 (26.8677, 0.1996) -> (27.1158, 0.0085) centre (30.2075, 4.2787) ccw
  arc A387 (27.1158, 0.0085) -> (27.4419, -0.2127) centre (30.8741, 5.1983) ccw
  arc A388 (27.4419, -0.2127) -> (27.8605, -0.4598) centre (31.5063, 6.1942) ccw
  arc A389 (27.8605, -0.4598) -> (28.1742, -0.2125) centre (15.3265, 15.7621) ccw
  arc A390 (28.1742, -0.2125) -> (28.0317, 0.2522) centre (20.853, -2.2042) ccw
  arc A391 (28.0317, 0.2522) -> (27.8927, 0.6209) centre (21.9689, -1.822) ccw
  arc A392 (27.8927, 0.6209) -> (27.7648, 0.9068) centre (23.0188, -1.3885) ccw
  arc A393 (27.7648, 0.9068) -> (28.0532, 1.1531) centre (15.3265, 15.7621) ccw
  arc A394 (28.0532, 1.1531) -> (28.3155, 0.982) centre (31.0626, 5.4816) ccw
  arc A395 (28.3155, 0.982) -> (28.6579, 0.7871) centre (31.655, 6.4507) ccw
  arc A396 (28.6579, 0.7871) -> (29.0946, 0.5736) centre (32.2071, 7.4931) ccw
  arc A397 (29.0946, 0.5736) -> (29.388, 0.8447) centre (15.3265, 15.7621) ccw
  arc A398 (29.388, 0.8447) -> (29.2094, 1.2969) centre (22.2456, -1.7153) ccw
  arc A399 (29.2094, 1.2969) -> (29.0419, 1.6535) centre (23.3281, -1.2466) ccw
  arc A400 (29.0419, 1.6535) -> (28.892, 1.9284) centre (24.3407, -0.7321) ccw
  arc A401 (28.892, 1.9284) -> (29.1602, 2.1966) centre (15.3265, 15.7621) ccw
  arc A402 (29.1602, 2.1966) -> (29.4351, 2.0467) centre (31.8207, 6.7479) ccw
  arc A403 (29.4351, 2.0467) -> (29.7917, 1.8792) centre (32.3352, 7.7605) ccw
  arc A404 (29.7917, 1.8792) -> (30.2439, 1.7006) centre (32.8039, 8.843) ccw
  arc A405 (30.2439, 1.7006) -> (30.515, 1.994) centre (15.3265, 15.7621) ccw
  arc A406 (30.515, 1.994) -> (30.3015, 2.4307) centre (23.5955, -1.1185) ccw
  arc A407 (30.3015, 2.4307) -> (30.1066, 2.7731) centre (24.6379, -0.5664) ccw
  arc A408 (30.1066, 2.7731) -> (29.9356, 3.0354) centre (25.607, 0.026) ccw
  arc A409 (29.9356, 3.0354) -> (30.1819, 3.3238) centre (15.3265, 15.7621) ccw
  arc A410 (30.1819, 3.3238) -> (30.4677, 3.1959) centre (32.4771, 8.0698) ccw
  arc A411 (30.4677, 3.1959) -> (30.8364, 3.057) centre (32.9106, 9.1197) ccw
  arc A412 (30.8364, 3.057) -> (31.3011, 2.9144) centre (33.2929, 10.2356) ccw
  arc A413 (31.3011, 2.9144) -> (31.5484, 3.2281) centre (15.3265, 15.7621) ccw
  arc A414 (31.5484, 3.2281) -> (31.3013, 3.6467) centre (24.8944, -0.4177) ccw
  arc A415 (31.3013, 3.6467) -> (31.0801, 3.9728) centre (25.8903, 0.2145) ccw
  arc A416 (31.0801, 3.9728) -> (30.889, 4.2209) centre (26.81, 0.8811) ccw
  arc A417 (30.889, 4.2209) -> (31.112, 4.5277) centre (15.3265, 15.7621) ccw
  arc A418 (31.112, 4.5277) -> (31.407, 4.4226) centre (33.0278, 9.4392) ccw
  arc A419 (31.407, 4.4226) -> (31.7854, 4.313) centre (33.3775, 10.5198) ccw
  arc A420 (31.7854, 4.313) -> (32.2599, 4.2073) centre (33.6711, 11.6623) ccw
  arc A421 (32.2599, 4.2073) -> (32.4818, 4.5395) centre (15.3265, 15.7621) ccw
  arc A422 (32.4818, 4.5395) -> (32.2026, 4.9374) centre (26.1344, 0.3829) ccw
  arc A423 (32.2026, 4.9374) -> (31.9566, 5.2451) centre (27.0776, 1.0913) ccw
  arc A424 (31.9566, 5.2451) -> (31.7466, 5.4775) centre (27.9421, 1.8279) ccw
  arc A425 (31.7466, 5.4775) -> (31.9447, 5.8008) centre (15.3265, 15.7621) ccw
  arc A426 (31.9447, 5.8008) -> (32.2471, 5.7192) centre (33.4693, 10.8475) ccw
  arc A427 (32.2471, 5.7192) -> (32.633, 5.6397) centre (33.7332, 11.9522) ccw
  arc A428 (32.633, 5.6397) -> (33.1143, 5.5715) centre (33.9362, 13.1142) ccw
  arc A429 (33.1143, 5.5715) -> (33.3095, 5.9201) centre (15.3265, 15.7621) ccw
  arc A430 (33.3095, 5.9201) -> (32.9999, 6.2949) centre (27.3077, 1.2782) ccw
  arc A431 (32.9999, 6.2949) -> (32.7304, 6.5823) centre (28.1924, 2.0585) ccw
  arc A432 (32.7304, 6.5823) -> (32.5029, 6.7975) centre (28.9965, 2.8607) ccw
  arc A433 (32.5029, 6.7975) -> (32.6751, 7.1354) centre (15.3265, 15.7621) ccw
  arc A434 (32.6751, 7.1354) -> (32.9829, 7.0777) centre (33.799, 12.2861) ccw
  arc A435 (32.9829, 7.0777) -> (33.3738, 7.0287) centre (33.9754, 13.4081) ccw
  arc A436 (33.3738, 7.0287) -> (33.859, 6.9986) centre (34.0866, 14.5825) ccw
  arc A437 (33.859, 6.9986) -> (34.0262, 7.3613) centre (15.3265, 15.7621) ccw
  arc A438 (34.0262, 7.3613) -> (33.6882, 7.7107) centre (28.4072, 2.2629) ccw
  arc A439 (33.6882, 7.7107) -> (33.397, 7.9761) centre (29.228, 3.1101) ccw
  arc A440 (33.397, 7.9761) -> (33.1533, 8.1727) centre (29.9666, 3.973) ccw
  arc A441 (33.1533, 8.1727) -> (33.2984, 8.5231) centre (15.3265, 15.7621) ccw
  arc A442 (33.2984, 8.5231) -> (33.6098, 8.4898) centre (34.0147, 13.7462) ccw
  arc A443 (33.6098, 8.4898) -> (34.0034, 8.4716) centre (34.1026, 14.8785) ccw
  arc A444 (34.0034, 8.4716) -> (34.4894, 8.4796) centre (34.1213, 16.058) ccw
  arc A445 (34.4894, 8.4796) -> (34.6277, 8.8544) centre (15.3265, 15.7621) ccw
  arc A446 (34.6277, 8.8544) -> (34.2633, 9.1762) centre (29.426, 3.3308) ccw
  arc A447 (34.2633, 9.1762) -> (33.9522, 9.4179) centre (30.1778, 4.2398) ccw
  arc A448 (33.9522, 9.4179) -> (33.6938, 9.5948) centre (30.8464, 5.158) ccw
  arc A449 (33.6938, 9.5948) -> (33.811, 9.9555) centre (15.3265, 15.7621) ccw
  arc A450 (33.811, 9.9555) -> (34.124, 9.9467) centre (34.1153, 15.2186) ccw
  arc A451 (34.124, 9.9467) -> (34.5178, 9.9594) centre (34.114, 16.3544) ccw
  arc A452 (34.5178, 9.9594) -> (35.0017, 10.0056) centre (34.0401, 17.5317) ccw
  arc A453 (35.0017, 10.0056) -> (35.1102, 10.39) centre (15.3265, 15.7621) ccw
  arc A454 (35.1102, 10.39) -> (34.7216, 10.6822) centre (30.3579, 4.4754) ccw
  arc A455 (34.7216, 10.6822) -> (34.3925, 10.8988) centre (31.036, 5.4406) ccw
  arc A456 (34.3925, 10.8988) -> (34.121, 11.0549) centre (31.6305, 6.4083) ccw
  arc A457 (34.121, 11.0549) -> (34.2096, 11.4237) centre (15.3265, 15.7621) ccw
  arc A458 (34.2096, 11.4237) -> (34.5223, 11.4395) centre (34.1, 16.6945) ccw
  arc A459 (34.5223, 11.4395) -> (34.9139, 11.4831) centre (34.0096, 17.8266) ccw
  arc A460 (34.9139, 11.4831) -> (35.3927, 11.567) centre (33.8436, 18.9945) ccw
  arc A461 (35.3927, 11.567) -> (35.4707, 11.9588) centre (15.3265, 15.7621) ccw
  arc A462 (35.4707, 11.9588) -> (35.0604, 12.2196) centre (31.1971, 5.6895) ccw
  arc A463 (35.0604, 12.2196) -> (34.7153, 12.4097) centre (31.7974, 6.7049) ccw
  arc A464 (34.7153, 12.4097) -> (34.4324, 12.544) centre (32.3142, 7.7164) ccw
  arc A465 (34.4324, 12.544) -> (34.4918, 12.9186) centre (15.3265, 15.7621) ccw
  arc A466 (34.4918, 12.9186) -> (34.8023, 12.9589) centre (33.969, 18.1645) ccw
  arc A467 (34.8023, 12.9589) -> (35.1893, 13.033) centre (33.7901, 19.2861) ccw
  arc A468 (35.1893, 13.033) -> (35.66, 13.1543) centre (33.5329, 20.4374) ccw
  arc A469 (35.66, 13.1543) -> (35.707, 13.551) centre (15.3265, 15.7621) ccw
  arc A470 (35.707, 13.551) -> (35.2775, 13.7788) centre (31.9384, 6.9657) ccw
  arc A471 (35.2775, 13.7788) -> (34.9186, 13.9413) centre (32.4572, 8.0251) ccw
  arc A472 (34.9186, 13.9413) -> (34.626, 14.053) centre (32.8931, 9.074) ccw
  arc A473 (34.626, 14.053) -> (34.6558, 14.431) centre (15.3265, 15.7621) ccw
  arc A474 (34.6558, 14.431) -> (34.9622, 14.4956) centre (33.723, 19.6198) ccw
  arc A475 (34.9622, 14.4956) -> (35.3421, 14.5999) centre (33.4566, 20.7239) ccw
  arc A476 (35.3421, 14.5999) -> (35.8019, 14.7577) centre (33.11, 21.8514) ccw
  arc A477 (35.8019, 14.7577) -> (35.8176, 15.1569) centre (15.3265, 15.7621) ccw
  arc A478 (35.8176, 15.1569) -> (35.3716, 15.3503) centre (32.5774, 8.2962) ccw
  arc A479 (35.3716, 15.3503) -> (35.0011, 15.4841) centre (33.0115, 9.3931) ccw
  arc A480 (35.0011, 15.4841) -> (34.7006, 15.5724) centre (33.3636, 10.4729) ccw
  arc A481 (34.7006, 15.5724) -> (34.7006, 15.9517) centre (15.3265, 15.7621) ccw
  arc A482 (34.7006, 15.9517) -> (35.0011, 16.0401) centre (33.3636, 21.0513) ccw
  arc A483 (35.0011, 16.0401) -> (35.3716, 16.1739) centre (33.0115, 22.1311) ccw
  arc A484 (35.3716, 16.1739) -> (35.8176, 16.3673) centre (32.5774, 23.2279) ccw
  arc A485 (35.8176, 16.3673) -> (35.8019, 16.7664) centre (15.3265, 15.7621) ccw
  arc A486 (35.8019, 16.7664) -> (35.3421, 16.9243) centre (33.11, 9.6727) ccw
  arc A487 (35.3421, 16.9243) -> (34.9622, 17.0286) centre (33.4566, 10.8002) ccw
  arc A488 (34.9622, 17.0286) -> (34.6558, 17.0931) centre (33.723, 11.9043) ccw
  arc A489 (34.6558, 17.0931) -> (34.626, 17.4712) centre (15.3265, 15.7621) ccw
  arc A490 (34.626, 17.4712) -> (34.9186, 17.5829) centre (32.8931, 22.4501) ccw
  arc A491 (34.9186, 17.5829) -> (35.2775, 17.7453) centre (32.4572, 23.499) ccw
  arc A492 (35.2775, 17.7453) -> (35.707, 17.9731) centre (31.9384, 24.5584) ccw
  arc A493 (35.707, 17.9731) -> (35.66, 18.3698) centre (15.3265, 15.7621) ccw
  arc A494 (35.66, 18.3698) -> (35.1893, 18.4911) centre (33.5329, 11.0868) ccw
  arc A495 (35.1893, 18.4911) -> (34.8023, 18.5653) centre (33.7901, 12.238) ccw
  arc A496 (34.8023, 18.5653) -> (34.4918, 18.6055) centre (33.969, 13.3596) ccw
  arc A497 (34.4918, 18.6055) -> (34.4324, 18.9801) centre (15.3265, 15.7621) ccw
  arc A498 (34.4324, 18.9801) -> (34.7153, 19.1144) centre (32.3142, 23.8078) ccw
  arc A499 (34.7153, 19.1144) -> (35.0604, 19.3045) centre (31.7974, 24.8192) ccw
  arc A500 (35.0604, 19.3045) -> (35.4707, 19.5653) centre (31.1971, 25.8346) ccw
  arc A501 (35.4707, 19.5653) -> (35.3927, 19.9571) centre (15.3265, 15.7621) ccw
  arc A502 (35.3927, 19.9571) -> (34.9139, 20.0411) centre (33.8436, 12.5296) ccw
  arc A503 (34.9139, 20.0411) -> (34.5223, 20.0847) centre (34.0096, 13.6975) ccw
  arc A504 (34.5223, 20.0847) -> (34.2096, 20.1005) centre (34.1, 14.8297) ccw
  arc A505 (34.2096, 20.1005) -> (34.121, 20.4692) centre (15.3265, 15.7621) ccw
  arc A506 (34.121, 20.4692) -> (34.3925, 20.6253) centre (31.6305, 25.1158) ccw
  arc A507 (34.3925, 20.6253) -> (34.7216, 20.8419) centre (31.036, 26.0836) ccw
  arc A508 (34.7216, 20.8419) -> (35.1102, 21.1341) centre (30.3579, 27.0488) ccw
  arc A509 (35.1102, 21.1341) -> (35.0017, 21.5186) centre (15.3265, 15.7621) ccw
  arc A510 (35.0017, 21.5186) -> (34.5178, 21.5647) centre (34.0401, 13.9924) ccw
  arc A511 (34.5178, 21.5647) -> (34.124, 21.5774) centre (34.114, 15.1697) ccw
  arc A512 (34.124, 21.5774) -> (33.811, 21.5686) centre (34.1153, 16.3055) ccw
  arc A513 (33.811, 21.5686) -> (33.6938, 21.9293) centre (15.3265, 15.7621) ccw
  arc A514 (33.6938, 21.9293) -> (33.9522, 22.1062) centre (30.8464, 26.3662) ccw
  arc A515 (33.9522, 22.1062) -> (34.2633, 22.348) centre (30.1778, 27.2843) ccw
  arc A516 (34.2633, 22.348) -> (34.6277, 22.6697) centre (29.426, 28.1933) ccw
  arc A517 (34.6277, 22.6697) -> (34.4894, 23.0445) centre (15.3265, 15.7621) ccw
  arc A518 (34.4894, 23.0445) -> (34.0034, 23.0525) centre (34.1213, 15.4661) ccw
  arc A519 (34.0034, 23.0525) -> (33.6098, 23.0343) centre (34.1026, 16.6456) ccw
  arc A520 (33.6098, 23.0343) -> (33.2984, 23.001) centre (34.0147, 17.778) ccw
  arc A521 (33.2984, 23.001) -> (33.1533, 23.3514) centre (15.3265, 15.7621) ccw
  arc A522 (33.1533, 23.3514) -> (33.397, 23.548) centre (29.9666, 27.5512) ccw
  arc A523 (33.397, 23.548) -> (33.6882, 23.8134) centre (29.228, 28.414) ccw
  arc A524 (33.6882, 23.8134) -> (34.0262, 24.1628) centre (28.4072, 29.2612) ccw
  arc A525 (34.0262, 24.1628) -> (33.859, 24.5256) centre (15.3265, 15.7621) ccw
  arc A526 (33.859, 24.5256) -> (33.3738, 24.4954) centre (34.0866, 16.9417) ccw
  arc A527 (33.3738, 24.4954) -> (32.9829, 24.4464) centre (33.9754, 18.116) ccw
  arc A528 (32.9829, 24.4464) -> (32.6751, 24.3888) centre (33.799, 19.238) ccw
  arc A529 (32.6751, 24.3888) -> (32.5029, 24.7267) centre (15.3265, 15.7621) ccw
  arc A530 (32.5029, 24.7267) -> (32.7304, 24.9418) centre (28.9965, 28.6635) ccw
  arc A531 (32.7304, 24.9418) -> (32.9999, 25.2293) centre (28.1924, 29.4657) ccw
  arc A532 (32.9999, 25.2293) -> (33.3095, 25.6041) centre (27.3077, 30.2459) ccw
  arc A533 (33.3095, 25.6041) -> (33.1143, 25.9526) centre (15.3265, 15.7621) ccw
  arc A534 (33.1143, 25.9526) -> (32.633, 25.8845) centre (33.9362, 18.4099) ccw
  arc A535 (32.633, 25.8845) -> (32.2471, 25.8049) centre (33.7332, 19.5719) ccw
  arc A536 (32.2471, 25.8049) -> (31.9447, 25.7233) centre (33.4693, 20.6766) ccw
  arc A537 (31.9447, 25.7233) -> (31.7466, 26.0467) centre (15.3265, 15.7621) ccw
  arc A538 (31.7466, 26.0467) -> (31.9566, 26.279) centre (27.9421, 29.6962) ccw
  arc A539 (31.9566, 26.279) -> (32.2026, 26.5867) centre (27.0776, 30.4329) ccw
  arc A540 (32.2026, 26.5867) -> (32.4818, 26.9846) centre (26.1344, 31.1413) ccw
  arc A541 (32.4818, 26.9846) -> (32.2599, 27.3168) centre (15.3265, 15.7621) ccw
  arc A542 (32.2599, 27.3168) -> (31.7854, 27.2111) centre (33.6711, 19.8618) ccw
  arc A543 (31.7854, 27.2111) -> (31.407, 27.1015) centre (33.3775, 21.0044) ccw
  arc A544 (31.407, 27.1015) -> (31.112, 26.9964) centre (33.0278, 22.085) ccw
  arc A545 (31.112, 26.9964) -> (30.889, 27.3033) centre (15.3265, 15.7621) ccw
  arc A546 (30.889, 27.3033) -> (31.0801, 27.5514) centre (26.81, 30.6431) ccw
  arc A547 (31.0801, 27.5514) -> (31.3013, 27.8774) centre (25.8903, 31.3096) ccw
  arc A548 (31.3013, 27.8774) -> (31.5484, 28.296) centre (24.8944, 31.9418) ccw
  arc A549 (31.5484, 28.296) -> (31.3011, 28.6097) centre (15.3265, 15.7621) ccw
  arc A550 (31.3011, 28.6097) -> (30.8364, 28.4672) centre (33.2929, 21.2885) ccw
  arc A551 (30.8364, 28.4672) -> (30.4677, 28.3282) centre (32.9106, 22.4045) ccw
  arc A552 (30.4677, 28.3282) -> (30.1819, 28.2003) centre (32.4771, 23.4543) ccw
  arc A553 (30.1819, 28.2003) -> (29.9356, 28.4887) centre (15.3265, 15.7621) ccw
  arc A554 (29.9356, 28.4887) -> (30.1066, 28.751) centre (25.607, 31.4982) ccw
  arc A555 (30.1066, 28.751) -> (30.3015, 29.0934) centre (24.6379, 32.0905) ccw
  arc A556 (30.3015, 29.0934) -> (30.515, 29.5302) centre (23.5955, 32.6427) ccw
  arc A557 (30.515, 29.5302) -> (30.2439, 29.8235) centre (15.3265, 15.7621) ccw
  arc A558 (30.2439, 29.8235) -> (29.7917, 29.6449) centre (32.8039, 22.6811) ccw
  arc A559 (29.7917, 29.6449) -> (29.4351, 29.4775) centre (32.3352, 23.7636) ccw
  arc A560 (29.4351, 29.4775) -> (29.1602, 29.3275) centre (31.8207, 24.7762) ccw
  arc A561 (29.1602, 29.3275) -> (28.892, 29.5957) centre (15.3265, 15.7621) ccw
  arc A562 (28.892, 29.5957) -> (29.0419, 29.8706) centre (24.3407, 32.2563) ccw
  arc A563 (29.0419, 29.8706) -> (29.2094, 30.2273) centre (23.3281, 32.7708) ccw
  arc A564 (29.2094, 30.2273) -> (29.388, 30.6794) centre (22.2456, 33.2394) ccw
  arc A565 (29.388, 30.6794) -> (29.0946, 30.9505) centre (15.3265, 15.7621) ccw
  arc A566 (29.0946, 30.9505) -> (28.6579, 30.737) centre (32.2071, 24.031) ccw
  arc A567 (28.6579, 30.737) -> (28.3155, 30.5421) centre (31.655, 25.0734) ccw
  arc A568 (28.3155, 30.5421) -> (28.0532, 30.3711) centre (31.0626, 26.0425) ccw
  arc A569 (28.0532, 30.3711) -> (27.7648, 30.6174) centre (15.3265, 15.7621) ccw
  arc A570 (27.7648, 30.6174) -> (27.8927, 30.9032) centre (23.0188, 32.9126) ccw
  arc A571 (27.8927, 30.9032) -> (28.0317, 31.2719) centre (21.9689, 33.3461) ccw
  arc A572 (28.0317, 31.2719) -> (28.1742, 31.7366) centre (20.853, 33.7284) ccw
  arc A573 (28.1742, 31.7366) -> (27.8605, 31.984) centre (15.3265, 15.7621) ccw
  arc A574 (27.8605, 31.984) -> (27.4419, 31.7368) centre (31.5063, 25.33) ccw
  arc A575 (27.4419, 31.7368) -> (27.1158, 31.5157) centre (30.8741, 26.3258) ccw
  arc A576 (27.1158, 31.5157) -> (26.8677, 31.3246) centre (30.2075, 27.2455) ccw
  arc A577 (26.8677, 31.3246) -> (26.5609, 31.5475) centre (15.3265, 15.7621) ccw
  arc A578 (26.5609, 31.5475) -> (26.666, 31.8425) centre (21.6494, 33.4633) ccw
  arc A579 (26.666, 31.8425) -> (26.7756, 32.2209) centre (20.5688, 33.8131) ccw
  arc A580 (26.7756, 32.2209) -> (26.8813, 32.6954) centre (19.4263, 34.1066) ccw
  arc A581 (26.8813, 32.6954) -> (26.5491, 32.9173) centre (15.3265, 15.7621) ccw
  arc A582 (26.5491, 32.9173) -> (26.1512, 32.6381) centre (30.7058, 26.5699) ccw
  arc A583 (26.1512, 32.6381) -> (25.8435, 32.3921) centre (29.9974, 27.5131) ccw
  arc A584 (25.8435, 32.3921) -> (25.6112, 32.1821) centre (29.2607, 28.3776) ccw
  arc A585 (25.6112, 32.1821) -> (25.2878, 32.3803) centre (15.3265, 15.7621) ccw
  arc A586 (25.2878, 32.3803) -> (25.3694, 32.6826) centre (20.2411, 33.9048) ccw
  arc A587 (25.3694, 32.6826) -> (25.449, 33.0685) centre (19.1364, 34.1687) ccw
  arc A588 (25.449, 33.0685) -> (25.5171, 33.5498) centre (17.9744, 34.3717) ccw
  arc A589 (25.5171, 33.5498) -> (25.1685, 33.745) centre (15.3265, 15.7621) ccw
  arc A590 (25.1685, 33.745) -> (24.7937, 33.4354) centre (29.8104, 27.7432) ccw
  arc A591 (24.7937, 33.4354) -> (24.5063, 33.166) centre (29.0302, 28.628) ccw
  arc A592 (24.5063, 33.166) -> (24.2911, 32.9384) centre (28.2279, 29.432) ccw
  arc A593 (24.2911, 32.9384) -> (23.9532, 33.1106) centre (15.3265, 15.7621) ccw
  arc A594 (23.9532, 33.1106) -> (24.0109, 33.4184) centre (18.8025, 34.2345) ccw